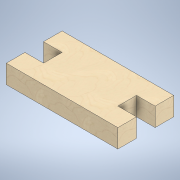
# Autodesk Inventor part: KabelBoxPlatteKurz
Saved by Autodesk Inventor 2020.3 (Build 243373010, 373A)
## iProperties
Created: 2021-02-15
Part Number: KabelBoxPlatteKurz
Material: Generisch
Document SubType Name: Modeling
Designer: Stefan
Density: 1 g/cm^3
Appearance: Pappel
Author: Stefan
Autodesk Inventor part; units mm, degrees
ref_plane "YZ Plane" through (0, 0, 0) normal (1, 0, 0) x (0, 1, 0)
ref_plane "XZ Plane" through (0, 0, 0) normal (0, 1, 0) x (-1, 0, 0)
ref_plane "XY Plane" through (0, 0, 0) normal (0, 0, 1) x (1, 0, 0)
sketch "Skizze1" plane through (0, 0, 0) normal (0, 1, 0) x (-1, 0, 0)
  line L0 (32.3571, 6.1813) -> (-27.6429, 6.1813)
  line L1 (-27.6429, -23.8187) -> (32.3571, -23.8187)
  line L2 (32.3571, -3.8187) -> (22.3571, -3.8187)
  line L3 (22.3571, -3.8187) -> (22.3571, -13.8187)
  line L4 (22.3571, -13.8187) -> (32.3571, -13.8187)
  line L5 (-17.6429, -3.8187) -> (-27.6429, -3.8187)
  line L6 (-27.6429, -13.8187) -> (-17.6429, -13.8187)
  line L7 (-17.6429, -13.8187) -> (-17.6429, -3.8187)
  line L8 (-27.6429, 6.1813) -> (-27.6429, -3.8187)
  line L9 (-27.6429, -13.8187) -> (-27.6429, -23.8187)
  line L10 (32.3571, -23.8187) -> (32.3571, -13.8187)
  line L11 (32.3571, -3.8187) -> (32.3571, 6.1813)
  point P0 (0, 0)
  dimension "d0" = 30
  dimension "d1" = 60
  dimension "d2" = 10
  dimension "d3" = 10
  dimension "d4" = 10
  dimension "d6" = 10
  dimension "d7" = 10
  dimension "d10" = 10
  constraints: 24 end point, 7 parallel, 3 horizontal, 3 perpendicular
  measures "d0" distance of L0.end L1.start
  measures "d1" distance of L0.start L0.end
  measures "d2" distance of L4.end L3.end
  measures "d3" distance of L3.end L2.end
  measures "d4" distance of L6.end L6.start
  measures "d6" distance between parallel lines of L0 L2
  measures "d7" distance between parallel lines of L0 L5
  measures "d10" distance of L6.end L5.start
extrude "Extrusion1" add sketch "Skizze1" along normal blind 10
